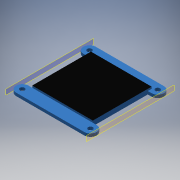
# Autodesk Inventor part: Pantalla
Saved by Autodesk Inventor 2019 (Build 230136000, 136)
## iProperties
Created: 2018-11-22
Part Number: Pantalla
Material: Steel, Mild, Welded
Document SubType Name: Modeling
Designer: cadcae
Density: 7.85 g/cm^3
Appearance: Cyan
Author: cadcae
Autodesk Inventor part; units mm, degrees
ref_plane "YZ Plane" through (0, 0, 0) normal (1, 0, 0) x (0, 1, 0)
ref_plane "XZ Plane" through (0, 0, 0) normal (0, 1, 0) x (-1, 0, 0)
ref_plane "XY Plane" through (0, 0, 0) normal (0, 0, 1) x (1, 0, 0)
sketch "Sketch1" plane through (0, 0, 0) normal (0, 1, 0) x (-1, 0, 0)
  line L0 (18, 22) -> (-18, 22)
  line L1 (-18, 15.5) -> (-16, 15.5)
  line L2 (-16, 15.5) -> (-16, -15.5)
  line L3 (-16, -13.5) -> (-18, -13.5)
  line L4 (-18, -20) -> (18, -20)
  line L5 (18, -13.5) -> (16, -13.5)
  line L6 (16, -15.5) -> (16, 15.5)
  line L7 (16, 15.5) -> (18, 15.5)
  arc A0 (-18, 22) -> (-18, 15.5) centre (-18, 18.75) ccw
  arc A1 (18, 15.5) -> (18, 22) centre (18, 18.75) ccw
  arc A2 (18, -20) -> (18, -13.5) centre (18, -16.75) ccw
  arc A3 (-18, -13.5) -> (-18, -20) centre (-18, -16.75) ccw
  line L8 (16, -15.5) -> (-16, -15.5)
  line L9 (-16, 15.5) -> (16, 15.5)
  circle A4 centre (18, -16.75) radius 1.25
  circle A5 centre (-18, -16.75) radius 1.25
  circle A6 centre (-18, 18.75) radius 1.25
  circle A7 centre (18, 18.75) radius 1.25
  point P0 (0, 0)
  point P1 (-3.7522, -13.5)
  point P2 (0, 22)
  point P3 (0, -20)
  point P4 (16, 0)
  point P5 (-16, 0)
  point P6 (0, -15.5)
  point P7 (0, 15.5)
  point P8 (0, 22)
  point P9 (-16, 0)
  dimension "d0" = 32
  dimension "d1" = 42
  dimension "d2" = 31
  dimension "d4" = 2.5
  dimension "d6" = 2
  dimension "d7" = 2
  constraints: 20 end point, 8 centre point, 8 midpoint, 8 point on circle, 8 tangent, 7 horizontal, 7 vertical alignment, 6 equal radius, 4 coincident, 4 point on line, 3 horizontal alignment, 2 parallel, 2 vertical
  measures "d0" distance between parallel lines of L2 L6
  measures "d1" distance between parallel lines of L0 L4
  measures "d2" distance between parallel lines of L9 L8
  measures "d4" diameter of A4
  measures "d6" radial gap between concentric circles of A0 A6
  measures "d7" distance from line of L2 A0.centre
extrude "Extrusion1" add sketch "Sketch1" against normal blind 1.57
extrude "Extrusion2" add sketch "Sketch1" along normal blind 1 contours L6 L8 L2 L9
ref_plane "Plano de trabajo1" through (21.25, 0, -16.75) normal (1, 0, 0) x (0, 0, -1)
ref_plane "Plano de trabajo2" through (-21.25, 0, -16.75) normal (-1, 0, 0) x (0, 0, 1)
body "Solid1"
